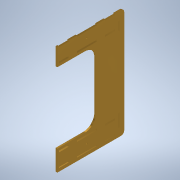
# Autodesk Inventor part: side bracer
Saved by Autodesk Inventor 2022 (Build 260153000, 153)
## iProperties
Created: 2021-05-28
Part Number: side bracer
Material: Brass, Soft Yellow
Document SubType Name: Modeling
Designer: benka
Density: 8.47 g/cm^3
Appearance: Brass - Satin
Author: benka
Autodesk Inventor part; units mm, degrees
ref_plane "YZ Plane" through (0, 0, 0) normal (1, 0, 0) x (0, 1, 0)
ref_plane "XZ Plane" through (0, 0, 0) normal (0, 1, 0) x (-1, 0, 0)
ref_plane "XY Plane" through (0, 0, 0) normal (0, 0, 1) x (1, 0, 0)
sketch "Sketch1" plane through (0, 0, 0) normal (1, 0, 0) x (0, 1, 0)
  line L0 (-181.2435, 115.0382) -> (-181.2435, -87.4618)
  line L1 (-80.2478, -7.4618) -> (73.7522, -7.4618)
  line L2 (-171.2435, -97.4618) -> (154.7524, -97.4618)
  line L3 (164.7524, -67.9618) -> (164.7524, -87.4618)
  circle A0 centre (141.7569, 21.2887) radius 2
  line L4 (-117.2477, 115.0382) -> (-181.2435, 115.0382)
  line L5 (-117.2477, 115.0382) -> (-115.2478, 115.0382)
  line L6 (-115.2478, 115.0382) -> (-115.2478, 27.5382)
  line L7 (108.7522, 27.5382) -> (108.7522, 115.0382)
  line L8 (108.7522, 115.0382) -> (164.7524, 115.0382)
  arc A1 (-181.2435, -87.4618) -> (-171.2435, -97.4618) centre (-171.2435, -87.4618) ccw
  line L9 (-128.2203, -67.9618) -> (-128.2203, -36.7118)
  line L10 (-128.2203, -36.7118) -> (-123.2203, -36.7118)
  line L11 (-123.2203, -67.9618) -> (-123.2203, -36.7118)
  line L12 (-128.2203, -67.9618) -> (-123.2203, -67.9618)
  line L13 (-128.2203, -10.4618) -> (-128.2203, 52.5382)
  line L14 (-128.2203, -10.4618) -> (-123.2203, -10.4618)
  line L15 (-123.2203, -10.4618) -> (-123.2203, 52.5382)
  line L16 (-128.2203, 52.5382) -> (-123.2203, 52.5382)
  line L17 (-128.2203, 78.7882) -> (-123.2203, 78.7882)
  line L18 (-123.2203, 78.7882) -> (-123.2203, 110.0382)
  line L19 (-128.2203, 110.0382) -> (-123.2203, 110.0382)
  line L20 (-128.2203, 78.7882) -> (-128.2203, 110.0382)
  circle A2 centre (-148.2261, 21.2878) radius 2
  line L21 (121.7524, 78.7882) -> (121.7524, 110.0382) projected
  line L22 (121.7524, 110.0382) -> (116.7524, 110.0382) projected
  line L23 (116.7524, 78.7882) -> (116.7524, 110.0382) projected
  line L24 (121.7524, 78.7882) -> (116.7524, 78.7882) projected
  line L25 (121.7524, -10.4618) -> (121.7524, 52.5382) projected
  line L26 (121.7524, 52.5382) -> (116.7524, 52.5382) projected
  line L27 (116.7524, -10.4618) -> (116.7524, 52.5382) projected
  line L28 (121.7524, -10.4618) -> (116.7524, -10.4618) projected
  line L29 (121.7524, -67.9618) -> (121.7524, -36.7118) projected
  line L30 (121.7524, -36.7118) -> (116.7524, -36.7118) projected
  line L31 (116.7524, -67.9618) -> (116.7524, -36.7118) projected
  line L32 (121.7524, -67.9618) -> (116.7524, -67.9618) projected
  line L33 (164.7524, 110.0382) -> (164.7524, 115.0382)
  line L34 (161.7524, 110.0382) -> (164.7524, 110.0382)
  line L35 (161.7524, 78.7882) -> (161.7524, 110.0382)
  line L36 (164.7524, 78.7882) -> (161.7524, 78.7882)
  line L37 (164.7524, 52.5382) -> (164.7524, 78.7882)
  line L38 (161.7524, 52.5382) -> (164.7524, 52.5382)
  line L39 (161.7524, -10.4618) -> (161.7524, 52.5382)
  line L40 (164.7524, -10.4618) -> (161.7524, -10.4618)
  line L41 (164.7524, -36.7118) -> (164.7524, -10.4618)
  line L42 (161.7524, -36.7118) -> (164.7524, -36.7118)
  line L43 (161.7524, -67.9618) -> (161.7524, -36.7118)
  line L44 (164.7524, -67.9618) -> (161.7524, -67.9618)
  arc A3 (73.7522, -7.4618) -> (108.7522, 27.5382) centre (73.7522, 27.5382) ccw
  arc A4 (-115.2478, 27.5382) -> (-80.2478, -7.4618) centre (-80.2478, 27.5382) ccw
  line L45 (-155.2478, -82.9618) -> (-115.2478, -82.9618) projected
  line L46 (-115.2478, -82.9618) -> (-115.2478, -77.9618) projected
  line L47 (-155.2478, -77.9618) -> (-115.2478, -77.9618) projected
  line L48 (-155.2478, -82.9618) -> (-155.2478, -77.9618) projected
  line L49 (108.7522, -82.9618) -> (138.0022, -82.9618) projected
  line L50 (138.0022, -82.9618) -> (138.0022, -77.9618) projected
  line L51 (108.7522, -77.9618) -> (138.0022, -77.9618) projected
  line L52 (108.7522, -82.9618) -> (108.7522, -77.9618) projected
  arc A5 (154.7524, -97.4618) -> (164.7524, -87.4618) centre (154.7524, -87.4618) ccw
  line L53 (-168.221, -67.9618) -> (-171.221, -67.9618)
  line L54 (-171.221, -36.7118) -> (-171.221, -67.9618)
  line L55 (-168.221, -36.7118) -> (-168.221, -67.9618)
  line L56 (-168.221, -36.7118) -> (-171.221, -36.7118)
  line L57 (-168.221, -10.4618) -> (-171.221, -10.4618)
  line L58 (-168.221, 52.5382) -> (-168.221, -10.4618)
  line L59 (-171.221, 52.5382) -> (-171.221, -10.4618)
  line L60 (-168.221, 52.5382) -> (-171.221, 52.5382)
  line L61 (-168.221, 78.7882) -> (-171.221, 78.7882)
  line L62 (-171.221, 110.0382) -> (-171.221, 78.7882)
  line L63 (-168.221, 110.0382) -> (-168.221, 78.7882)
  line L64 (-168.221, 110.0382) -> (-171.221, 110.0382)
  point P0 (141.7524, 19.2994)
  point P1 (143.3399, 20.8869)
  point P2 (164.7524, -92.4608)
  point P3 (161.7524, -97.4618)
  point P4 (-176.2435, -97.4618)
  point P5 (-181.2435, -92.4608)
  point P6 (-115.2478, 7.8284)
  point P7 (-107.2347, -7.4618)
  point P8 (98.7522, -7.4618)
  point P9 (108.7522, 9.8153)
  point P10 (156.7524, -97.4618)
  point P11 (-95.2478, -7.4618)
  point P12 (-115.2478, 12.5382)
  dimension "d40" = 212.5
  dimension "d41" = 212.5
  dimension "d44" = 4
  dimension "d50" = 35
  dimension "d51" = 90
  dimension "d52" = 35
  dimension "d54" = 3
  dimension "d55" = 10
  constraints: 90 end point, 14 horizontal, 14 vertical, 12 point on line, 11 collinear, 8 point on circle, 8 tangent, 6 centre point, 2 parallel, 1 perpendicular, 26 other
  measures "d40" distance between parallel lines of L2 L8
  measures "d41" distance between parallel lines of L2 L4
  measures "d44" diameter of A2
  measures "d50" radius of A3
  measures "d51" distance between parallel lines of L2 L1
  measures "d52" radius of A4
  measures "d54" distance between parallel lines of L35 L33
  measures "d55" radius of A5
extrude "Extrusion1" add sketch "Sketch1" along normal blind 5
body "Solid1"
